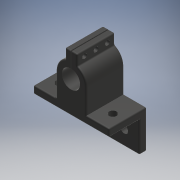
# Autodesk Inventor part: z_rod_holder
Saved by Autodesk Inventor 2018 (Build 220112000, 112)
## iProperties
Created: 2018-05-26
Part Number: z_rod_holder
Material: Plastic, Opaque Black
Document SubType Name: Modeling
Designer: Z. Deniz
Density: 0.952 g/cm^3
Appearance: Smooth - Black
Author: Z. Deniz
Autodesk Inventor part; units mm, degrees
ref_plane "YZ Plane" through (0, 0, 0) normal (1, 0, 0) x (0, 1, 0)
ref_plane "XZ Plane" through (0, 0, 0) normal (0, 1, 0) x (-1, 0, 0)
ref_plane "XY Plane" through (0, 0, 0) normal (0, 0, 1) x (1, 0, 0)
sketch "Sketch1" plane through (0, 0, 0) normal (0, 1, 0) x (-1, 0, 0)
  line L0 (25, -12.5) -> (-25, -12.5)
  line L1 (-25, -12.5) -> (-25, 12.5)
  line L2 (-25, 12.5) -> (25, 12.5)
  line L3 (25, 12.5) -> (25, -12.5)
  line L4 (25, -12.5) -> (-25, 12.5) construction
  line L5 (-25, -12.5) -> (25, 12.5) construction
  arc A0 (-3.3467, 33.4799) -> (-4, 32.9721) centre (0, 28.5) ccw
  arc A1 (-4, 37.6652) -> (4, 37.6652) centre (0, 28.5) ccw
  line L6 (25, -12.5) -> (-25, -12.5)
  line L7 (-25, -12.5) -> (-25, 7.5)
  line L8 (-25, 7.5) -> (25, 7.5)
  line L9 (25, 7.5) -> (25, -12.5)
  line L10 (0, 28.5) -> (0, 0) construction
  line L11 (10, 28.5) -> (10, 12.5)
  line L12 (-10, 28.5) -> (-10, 12.5)
  line L13 (-4, 44.5) -> (-0.3, 44.5)
  line L14 (4, 44.5) -> (4, 37.6652)
  line L15 (4, 32.5) -> (-4, 32.5) construction
  line L16 (-4, 32.5) -> (-4, 32.9721) construction
  line L17 (-4, 44.5) -> (4, 32.5) construction
  line L18 (4, 44.5) -> (-4, 32.5) construction
  line L19 (0, 28.5) -> (0, 38.5) construction
  line L20 (-4, 37.6652) -> (-4, 44.5)
  line L21 (4, 37.6652) -> (4, 32.9721) construction
  line L22 (4, 32.9721) -> (4, 32.5) construction
  line L23 (-4, 32.9721) -> (-4, 37.6652) construction
  arc A2 (0, 38.5) -> (-4, 37.6652) centre (0, 28.5) ccw construction
  arc A3 (4, 37.6652) -> (0, 38.5) centre (0, 28.5) ccw construction
  arc A4 (0, 34.5) -> (-0.3, 34.4925) centre (0, 28.5) ccw construction
  arc A5 (-4, 32.9721) -> (4, 32.9721) centre (0, 28.5) ccw
  arc A6 (3.3467, 33.4799) -> (0.3, 34.4925) centre (0, 28.5) ccw
  arc A7 (4, 32.9721) -> (3.3467, 33.4799) centre (0, 28.5) ccw
  line L24 (0.3, 44.5) -> (0.3, 34.4925)
  line L25 (-0.3, 44.5) -> (-0.3, 34.4925)
  line L26 (0.3, 44.5) -> (4, 44.5)
  line L27 (-0.3, 44.5) -> (0.3, 44.5) construction
  arc A8 (0.3, 34.4925) -> (0, 34.5) centre (0, 28.5) ccw construction
  arc A9 (-0.3, 34.4925) -> (-3.3467, 33.4799) centre (0, 28.5) ccw
  line L28 (25, -12.5) -> (-25, 7.5) construction
  line L29 (-25, -12.5) -> (25, 7.5) construction
  line L30 (25, -2.5) -> (0, -2.5) construction
  line L31 (0, -2.5) -> (-25, -2.5) construction
  circle A10 centre (0, -2.5) radius 2.5
  circle A11 centre (15, -2.5) radius 2.5
  circle A12 centre (-15, -2.5) radius 2.5
  dimension "d1" = 25
  dimension "d3" = 20
  dimension "d5" = 20
  dimension "d6" = 21
  dimension "d7" = 50
  dimension "d8" = 8
  dimension "d9" = 12
  dimension "d10" = 0.3
  dimension "d12" = 0.3
  dimension "d13" = 6
  dimension "d18" = 5
  dimension "d19" = 5
  dimension "d20" = 5
  dimension "d21" = 10
  dimension "d22" = 10
  constraints: 64 end point, 26 point on circle, 16 parallel, 16 perpendicular, 13 centre point, 8 point on line, 7 midpoint, 5 horizontal, 4 tangent, 3 vertical, 2 coincident
  measures "d1" distance of L0.end L1.end
  measures "d3" diameter of A1
  measures "d5" distance of L6.end L7.end
  measures "d6" distance from line of A0.centre L8
  measures "d7" distance between parallel lines of L7 L3
  measures "d8" distance of L15.start L15.end
  measures "d9" distance of L14.start L15.start
  measures "d10" distance between parallel lines of L24 L19
  measures "d12" distance between parallel lines of L25 L19
  measures "d13" radius of A5
  measures "d18" diameter of A10
  measures "d19" diameter of A11
  measures "d20" diameter of A12
  measures "d21" distance from line of L9 A11.centre
  measures "d22" distance from line of L7 A12.centre
extrude "Extrusion1" add sketch "Sketch1" against normal blind 5 contours L0 L1 L8 L3
extrude "Extrusion2" add sketch "Sketch1" against normal blind 25 contours L8 L1 L2 L3 | L2 L12 A1 L11 | A1 L20 L13 L25 A9 A0 A5 A7 A6 L24 L26 L14
sketch "Sketch2" plane through (25, -5, 7.5) normal (0, 0, -1) x (-1, 0, 0)
  line L0 (0, -20) -> (15, -20) projected
  line L1 (50, 0) -> (0, 0)
  line L2 (0, 0) -> (0, -20)
  line L3 (0, -20) -> (50, -20)
  line L4 (50, -20) -> (50, 0)
  line L5 (0, 5) -> (0, -20) construction
  line L6 (0, -10) -> (50, -10) construction
  circle A0 centre (7.5, -10) radius 2.5
  circle A1 centre (42.5, -10) radius 2.5
  point P0 (25, 5)
  dimension "d26" = 5
  dimension "d27" = 7.5
  dimension "d28" = 5
  dimension "d29" = 7.5
  constraints: 10 end point, 3 point on line, 2 centre point, 2 parallel, 1 horizontal, 1 midpoint, 1 perpendicular
  measures "d26" diameter of A0
  measures "d27" distance from line of L2 A0.centre
  measures "d28" diameter of A1
  measures "d29" distance from line of L4 A1.centre
extrude "Extrusion3" cut sketch "Sketch2" against normal blind 5 contours A0 | A1
sketch "Sketch3" plane through (4, 0, 44.5) normal (1, 0, 0) x (0, 0, -1)
  line L0 (0, 0) -> (0, -25) construction
  line L1 (6.8348, 0) -> (6.8348, -25) construction
  line L2 (0, 0) -> (6.8348, 0) construction
  line L3 (6.8348, 0) -> (6.8348, -25) construction
  line L4 (6.8348, -25) -> (0, -25) construction
  line L5 (0, -25) -> (0, 0) construction
  line L6 (6.8348, -25) -> (0, -25) construction
  line L7 (0, 0) -> (6.8348, -25) construction
  line L8 (0, 0) -> (6.8348, 0) construction
  line L9 (0, -25) -> (6.8348, 0) construction
  line L10 (3.4174, 0) -> (3.4174, -12.5) construction
  line L11 (3.4174, -12.5) -> (3.4174, -25) construction
  circle A0 centre (3.4174, -12.5) radius 1.575
  circle A1 centre (3.4174, -5) radius 1.575
  circle A2 centre (3.4174, -20) radius 1.575
  point P0 (44.5, 0)
  dimension "d32" = 3.15
  dimension "d33" = 3.15
  dimension "d34" = 3.15
  dimension "d35" = 5
  dimension "d36" = 5
  constraints: 16 end point, 3 centre point, 3 midpoint, 2 parallel, 2 point on line, 1 coincident, 1 horizontal, 1 perpendicular
  measures "d32" diameter of A0
  measures "d33" diameter of A1
  measures "d34" diameter of A2
  measures "d35" distance from line of L4 A2.centre
  measures "d36" distance from line of L2 A1.centre
extrude "Extrusion4" cut sketch "Sketch3" against normal blind 8
fillet "Fillet1" radius 1 40 edges at (-25, -12.5, 12.5) (-25, -15, 7.5) (-25, -5, -2.5) (-25, 0, 0) (-17.5, 0, 12.5) (-8.3666, 0, 33.9772) (-10, 0, 20.5) (-10, -12.5, 12.5) (-4, -12.5, 37.6652) (-4, 0, 41.0826) (-4, -12.5, 44.5) (-4, -25, 41.0826) (-10, -25, 20.5) (-8.3666, -25, 33.9772) (-17.5, -25, 12.5) (0, -25, 7.5) (-2.15, 0, 44.5) (2.15, 0, 44.5) (4, 0, 41.0826) (10, 0, 20.5) (8.3666, 0, 33.9772) (10, -25, 20.5) (8.3666, -25, 33.9772) (-2.15, -25, 44.5) (2.15, -25, 44.5) (4, -12.5, 44.5) (4, -25, 41.0826) (17.5, -25, 12.5) (25, -12.5, 12.5) (17.5, 0, 12.5) (25, 0, 0) (0, 0, -12.5) (25, -2.5, -12.5) (0, -5, -12.5) (25, -5, -2.5) (25, -15, 7.5) (25, -25, 10) (-25, -2.5, -12.5) (-25, -25, 10) (4, -12.5, 37.6652)
body "Solid1"
